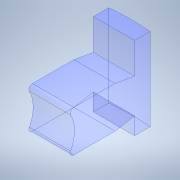
# Autodesk Inventor part: shank_2
Saved by Autodesk Inventor 2020.2 (Build 242310000, 310)
## iProperties
Created: 2021-01-30
Part Number: shank_2
Material: Generic
Document SubType Name: Modeling
Designer: DELL
Density: 1 g/cm^3
Appearance: Clear - Blue
Author: DELL
Autodesk Inventor part; units mm, degrees
ref_plane "YZ Plane" through (0, 0, 0) normal (1, 0, 0) x (0, 1, 0)
ref_plane "XZ Plane" through (0, 0, 0) normal (0, 1, 0) x (-1, 0, 0)
ref_plane "XY Plane" through (0, 0, 0) normal (0, 0, 1) x (1, 0, 0)
sketch "Sketch17" plane through (0, 0, 0) normal (1, 0, 0) x (0, 1, 0)
  line L0 (-67.9, 0) -> (67.9, 0) construction
  line L1 (0, -67.9) -> (0, 67.9) construction
  circle A0 centre (0, 0) radius 40
  circle A1 centre (0, 0) radius 48.5
  dimension "d173" = 97
  dimension "d174" = 80
  constraints: 2 centre point, 2 coincident
  measures "d173" diameter of A1
  measures "d174" diameter of A0
sketch "Sketch16" plane through (0, 0, 0) normal (1, 0, 0) x (0, 1, 0)
  circle A0 centre (0, 0) radius 40
  circle A1 centre (0, 0) radius 48.5
  line L0 (0, -201.7) -> (0, 90.2) construction
  line L1 (0, -160) -> (0, -48.5)
  line L2 (30, -38.1084) -> (30, -107.6436)
  line L3 (30, -107.6436) -> (25, -136)
  line L4 (25, -136) -> (50, -136)
  line L5 (50, -136) -> (50, -160)
  line L6 (50, -160) -> (0, -160)
  dimension "d156" = 97
  dimension "d157" = 80
  dimension "d202" = 24
  dimension "d203" = 60
  dimension "d204" = 50
  dimension "d206" = 160
  dimension "d209" = 50
  dimension "d210" = 80
  dimension "d211" = 28.7938
  constraints: 12 end point, 2 centre point, 2 coincident, 2 horizontal, 2 point on circle, 2 point on line, 2 vertical
  measures "d156" diameter of A1
  measures "d157" diameter of A0
  measures "d202" distance of L4.end L5.end
  measures "d203" diameter of L2 L0
  measures "d204" distance of L5.end L1.start
  measures "d206" distance from line of point (0, 0) L6
  measures "d209" diameter of L3.end L0
  measures "d210" angle of L4 L3
  measures "d211" distance of L2.end L3.end
extrude "Extrusion14" add sketch "Sketch16" along normal mid plane 60 contours A1 L2 L3 L4 L5 L6 L1
fillet "Fillet10" radius 5 1 edges at (0, 30, -38.1084)
mirror "Mirror1" about plane through (0, 0, 0) normal (0, 1, 0)
thicken "Thicken1" operation add thickness 20 both sides no extend neighbours yes toward (0, 1, 0) faces at (10, 50, -152)
sketch "Sketch19" plane through (0, 0, 0) normal (0, 1, 0) x (-1, 0, 0)
  arc A0 (-141.325, -124.6266) -> (141.325, -124.6266) centre (0, 140) ccw
  line L0 (164.3666, 0) -> (-121.2598, 0) projected
  line L1 (0, -205.7584) -> (0, 90.8764) projected
  line L2 (141.325, -124.6266) -> (141.325, -203.0263)
  line L3 (141.325, -203.0263) -> (-141.325, -202.4208)
  line L4 (-141.325, -202.4208) -> (-141.325, -124.6266)
  point P0 (0, 0)
  point P1 (0, -160)
  point P2 (0, -160)
  dimension "d217" = 300
  dimension "d218" = 0
  constraints: 6 end point, 3 point on circle, 2 point on line, 2 vertical, 1 centre point, 1 symmetric about line
  measures "d217" radius of A0
  measures "d218" distance of point (0, -160) point (0, -160)
extrude "Extrusion16" cut sketch "Sketch19" along normal through all both and the other way through all
body "Solid1"
body "Solid6"
